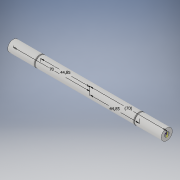
# Autodesk Inventor part: Auspressrolle
Saved by Autodesk Inventor 2018 (Build 220112000, 112)
## iProperties
Created: 2018-01-12
Part Number: Auspressrolle
Material: Generisch
Document SubType Name: Modeling
Designer: Julian
Density: 1 g/cm^3
Appearance: Vorgabe
Author: Julian
Autodesk Inventor part; units mm, degrees
ref_plane "YZ Plane" through (0, 0, 0) normal (1, 0, 0) x (0, 1, 0)
ref_plane "XZ Plane" through (0, 0, 0) normal (0, 1, 0) x (-1, 0, 0)
ref_plane "XY Plane" through (0, 0, 0) normal (0, 0, 1) x (1, 0, 0)
sketch "Skizze1" plane through (0, 0, 0) normal (1, 0, 0) x (0, 1, 0)
  circle A0 centre (0, 0) radius 5
  dimension "d0" = 10
  constraints: 1 centre point, 1 coincident
  measures "d0" diameter of A0
extrude "Extrusion1" add sketch "Skizze1" along normal blind 140
sketch "Skizze2" plane through (0, 0, 0) normal (-1, 0, 0) x (0, 0, 1)
  point P0 (0, 0)
  point P1 (0, 0)
  constraints: 1 coincident
hole "Bohrung1" at (0, 0, 0) direction (1, 0, 0) diameter 4.134 depth 14.2 tip angle 118 thread size "M5x0.8" class "6H" standard "ISO Metric profile"
sketch "Skizze3" plane through (140, 0, 0) normal (1, 0, 0) x (0, 0, -1)
  point P0 (0, 0)
  point P1 (0, 0)
  constraints: 1 coincident
hole "Bohrung2" at (140, 0, 0) direction (-1, 0, 0) diameter 4.134 depth 14.2 tip angle 118 thread size "M5x0.8" class "6H" standard "ISO Metric profile"
sketch "Skizze4" plane through (0, 0, 0) normal (0, 1, 0) x (-1, 0, 0)
  line L0 (0, 0) -> (-70, 0)
  line L1 (-70, 0) -> (-140, 0)
  line L2 (-140, -2.067) -> (-140, 2.067) projected
  line L3 (-70, 0) -> (-114.85, 0)
  line L4 (-70, 0) -> (-25.15, 0)
  dimension "d17" = 70
  dimension "d18" = 70
  dimension "d19" = 44.85
  dimension "d23" = 44.85
  constraints: 8 end point, 2 point on line, 1 horizontal, 1 midpoint
  measures "d17" distance of L0.start L0.end
  measures "d18" distance of L0.end L1.end
  measures "d19" distance of L0.end L3.end
  measures "d23" distance of L0.end L4.end
ref_plane "Arbeitsebene1" through (114.85, 0, 0) normal (1, 0, 0) x (0, 1, 0)
sketch "Skizze5" plane through (114.85, 0, 0) normal (1, 0, 0) x (0, 1, 0)
  circle A0 centre (0, 0) radius 5
  circle A1 centre (0, 0) radius 4
  dimension "d20" = 8
  constraints: 2 centre point, 2 coincident
  measures "d20" diameter of A1
extrude "Extrusion2" cut sketch "Skizze5" along normal blind 0.9
ref_plane "Arbeitsebene2" through (25.15, 0, 0) normal (1, 0, 0) x (0, 1, 0)
sketch "Skizze6" plane through (25.15, 0, 0) normal (1, 0, 0) x (0, 1, 0)
  circle A0 centre (0, 0) radius 5
  circle A1 centre (0, 0) radius 4
  dimension "d24" = 8
  constraints: 2 centre point, 2 coincident
  measures "d24" diameter of A1
extrude "Extrusion3" cut sketch "Skizze6" against normal blind 0.9
